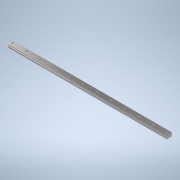
# Autodesk Inventor part: 02_mgn15h_Rail_450mm
Saved by Autodesk Inventor 2022.2 (Build 262287010, 287A)
## iProperties
Created: 2022-03-20
Part Number: 02_mgn15h_Rail_450mm
Material: Edelstahl
Document SubType Name: Modeling
Designer: MXBD
Density: 8 g/cm^3
Appearance: Halbpoliert
Mass: 495.656 g
Surface Area: 254.488 cm^2
Volume: 61.957 cm^3
Author: MXBD
Autodesk Inventor part; units mm, degrees
ref_plane "YZ Plane" through (0, 0, 0) normal (1, 0, 0) x (0, 1, 0)
ref_plane "XZ Plane" through (0, 0, 0) normal (0, 1, 0) x (-1, 0, 0)
ref_plane "XY Plane" through (0, 0, 0) normal (0, 0, 1) x (1, 0, 0)
sketch "Skizze1" plane through (0, 0, 0) normal (1, 0, 0) x (0, 1, 0)
  line L0 (0, 0) -> (0, -7.5)
  line L1 (0, -7.5) -> (5, -7.5)
  line L2 (0, -10.5) -> (0, 10.5) projected
  line L3 (-2, 0) -> (12, 0) projected
  arc A0 (8, -7.5) -> (5, -7.5) centre (6.5, -7.5) ccw
  line L4 (8, -7.5) -> (10, -7.5)
  line L5 (10, -7.5) -> (10, 0)
  line L6 (0, 0) -> (0, 7.5)
  line L7 (0, 7.5) -> (5, 7.5)
  arc A1 (5, 7.5) -> (8, 7.5) centre (6.5, 7.5) ccw
  line L8 (8, 7.5) -> (10, 7.5)
  line L9 (10, 7.5) -> (10, 0)
  dimension "d1" = 1.5
  dimension "d2" = 15
  dimension "d3" = 10
  dimension "d4" = 3.5
  constraints: 17 end point, 6 point on line, 6 symmetric about line, 4 point on circle, 2 centre point, 2 perpendicular, 1 horizontal, 1 vertical, 1 other
  measures "d1" radius of A0
  measures "d2" distance between parallel lines of L1 L7
  measures "d3" distance between parallel lines of L5 L0
  measures "d4" distance from line of L5 A0.centre
extrude "Extrusion1" add sketch "Skizze1" along normal mid plane 450
chamfer "Fase1" distance 0.4 distance2 0.4 2 edges at (0, 10, 7.5) (0, 10, -7.5) measured on face at (75, 8.6667, -7.5) measured on face at (75, 10, 2.5)
chamfer "Fase2" distance 0.4 distance2 0.4 1 edges at (0, 0, 7.5) measured on face at (-75, 3.3333, 7.5)
chamfer "Fase3" distance 0.4 distance2 0.4 1 edges at (0, 0, -7.5) measured on face at (-75, 1.6667, -7.5)
sketch "Skizze2" plane through (-225, 10, -7.1) normal (0, 1, 0) x (1, 0, 0)
  line L0 (-90, -7.1) -> (540, -7.1) projected
  line L1 (450, 0) -> (450, -14.2) projected
  point P0 (225, -7.1)
  point P1 (445, -7.1)
  dimension "d16" = 5
  constraints: 1 point on line
  measures "d16" distance from line of point (445, -7.1) L1
hole "Bohrung1" at (220, 10, 0) direction (0, -1, 0) diameter 3.4 end through all counterbore diameter 6 counterbore depth 4.9 clearance for "Inbusschraube DIN EN ISO 4762" size "M3" standard "DIN"
pattern_linear "Rechteckige Anordnung1" count 12 spacing 40 along (-1, 0, 0) of "Bohrung1"
